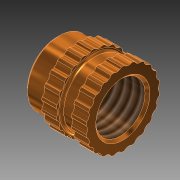
# Autodesk Inventor part: Втулка 2
Saved by Autodesk Inventor 2021.3 (Build 253353000, 353)
## iProperties
Part Number: Втулка 2
Checked By: Якушев
Engr Approved By: Малов
Material: По умолчанию1
Document SubType Name: Modeling
Mfg Approved By: Судаков
Designer: Смирнов
Density: 1 g/cm^3
Appearance: Металл — 1600F
RuleStatus: InUse
AfterMaterialChange0: Материал
BeforeDocSave0: Материал
AfterAnyiPropertyChange0: Материал
Author: Смирнов
Материал: По умолчанию1
Autodesk Inventor part; units mm, degrees
ref_plane "YZ Plane" through (0, 0, 0) normal (1, 0, 0) x (0, 1, 0)
ref_plane "XZ Plane" through (0, 0, 0) normal (0, 1, 0) x (-1, 0, 0)
ref_plane "XY Plane" through (0, 0, 0) normal (0, 0, 1) x (1, 0, 0)
sketch "Эскиз1" plane through (0, 0, 0) normal (0, 0, 1) x (1, 0, 0)
  line L0 (0, 0) -> (0, 22.3165) construction
  line L1 (0, 0) -> (21.2367, 0) construction
  line L2 (-4, 1.95) -> (-2.7, 1.95)
  line L3 (-2.7, 1.95) -> (-2.7, 2.25)
  line L4 (-2.7, 2.25) -> (-1.8, 2.25)
  line L5 (-1.8, 2.25) -> (-1.8, 1.95)
  line L6 (-1.8, 1.95) -> (-0.9, 1.95)
  line L7 (-0.9, 1.95) -> (-0.9, 2.25)
  line L8 (-0.9, 2.25) -> (0, 2.25)
  line L9 (0, 2.25) -> (0, 1.5)
  line L10 (0, 1.5) -> (-4, 1.5)
  line L11 (-4, 1.5) -> (-4, 1.95)
  dimension "d0" = 3
  dimension "d1" = 4.5
  dimension "d2" = 4
  dimension "d3" = 0.9
  dimension "d4" = 0.3
  constraints: 24 end point, 6 perpendicular, 3 vertical, 2 collinear, 2 equal length, 2 horizontal, 2 point on line
  measures "d0" diameter of L10 L1
  measures "d1" diameter of L4 L1
  measures "d2" distance between parallel lines of L11 L0
  measures "d3" distance of L7.end L8.end
  measures "d4" distance between parallel lines of L8 L6
revolve "Вращение1" add sketch "Эскиз1" angle 360 about axis through (0, 0, 0) along (1, 0, 0)
sketch "Эскиз2" plane through (0, 0, 0) normal (1, 0, 0) x (0, 0, -1)
  line L0 (0, 0) -> (0, 3.5465) construction
  circle A0 centre (0, 0) radius 2.25 construction
  circle A1 centre (0, 2.5) radius 0.35
  dimension "d6" = 0.7
  dimension "d7" = 2.5
  constraints: 2 end point, 1 centre point, 1 point on line, 1 vertical
  measures "d6" diameter of A1
  measures "d7" distance of A1.centre L0.start
extrude "Выдавливание1" cut sketch "Эскиз2" against normal blind 10
pattern_circular "Круговой массив1" count 22 over 360 about axis through (-10, 0, 0) along (1, 0, 0) of "Выдавливание1"
thread "Резьба1" size "M3x0.5" class "6H" standard "ANSI Metric M Profile" full length
chamfer "Фаска1" distance 0.15 angle 45 3 edges at (0, -1.5, 0) (-4, -1.5, 0) (-4, -1.95, 0)
fillet "Сопряжение1" radius 0.15 3 edges at (-1.8, -1.95, 0) (-0.9, -1.95, 0) (-2.7, -1.95, 0)
